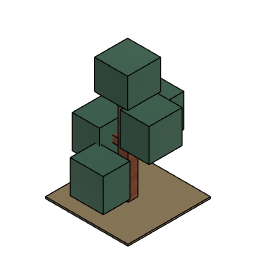
Tree v3 (Autodesk Fusion 360 design; units mm, degrees)
Autodesk Fusion 360 part; units mm, degrees
sketch "Skizze1" plane through (0, 0, 0) normal (0, 0, 1) x (1, 0, 0)
  line L0 (0, 0) -> (50, 0)
  line L1 (50, 0) -> (50, 50)
  line L2 (50, 50) -> (0, 50)
  line L3 (0, 50) -> (0, 0)
  line L4 (0, 25) -> (50, 25) construction
  line L5 (25, 50) -> (25, 0) construction
  constraint coincident L0.start L3.end
  constraint midpoint L3 L4.start
  constraint midpoint L1 L4.end
  constraint midpoint L2 L5.start
  constraint midpoint L0 L5.end
  constraint perpendicular L0 L5
extrude "Extrusion1" add sketch "Skizze1" against normal blind 1 makes body 1 in component "Ground"
ref_plane "Arbeitsebene1" through (25, 25, 0) normal (0, -1, 0) x (1, 0, 0)
ref_plane "Arbeitsebene2" through (25, 25, 0) normal (-1, 0, 0) x (0, -1, 0)
sketch "Skizze2" plane through (25, 25, 0) normal (0, -1, 0) x (1, 0, 0)
  line L0 (-25, 0) -> (25, 0)
  line L1 (0, 0) -> (0, 75) construction
  line L2 (-3, 0) -> (-3, 65)
  line L3 (-3, 65) -> (3, 65)
  line L4 (3, 65) -> (3, 0)
  line L5 (-3, 0) -> (3, 0)
  line L6 (-3, 29.6581) -> (-20.0867, 29.6581)
  line L7 (-20.0867, 29.6581) -> (-20.0867, 25.6581)
  line L8 (-20.0867, 25.6581) -> (-3, 25.6581)
  line L9 (-3, 25.6581) -> (-3, 29.6581)
  line L10 (3, 44.9151) -> (20.4397, 44.9151)
  line L11 (20.4397, 44.9151) -> (20.4397, 40.9151)
  line L12 (20.4397, 40.9151) -> (3, 40.9151)
  line L13 (3, 40.9151) -> (3, 44.9151)
  line L14 (-23.7757, 37.2774) -> (-7.2473, 37.2774)
  line L15 (-7.2473, 37.2774) -> (-7.2473, 17.2774)
  line L16 (-7.2473, 17.2774) -> (-23.7757, 17.2774)
  line L17 (-23.7757, 17.2774) -> (-23.7757, 37.2774)
  line L18 (5.3079, 53.1701) -> (22.7898, 53.1701)
  line L19 (22.7898, 53.1701) -> (22.7898, 33.1701)
  line L20 (22.7898, 33.1701) -> (5.3079, 33.1701)
  line L21 (5.3079, 33.1701) -> (5.3079, 53.1701)
  line L22 (-10.267, 73.036) -> (9.733, 73.036)
  line L23 (9.733, 73.036) -> (9.733, 55)
  line L24 (9.733, 55) -> (-10.267, 55)
  line L25 (-10.267, 55) -> (-10.267, 73.036)
  dimension "d21" = 6
  dimension "d25" = 3
  dimension "d26" = 4
  dimension "d27" = 4
  dimension "d36" = 20
  dimension "d37" = 20
  dimension "d38" = 20
  constraint coincident L1.start origin
  constraint perpendicular L0 L1
  constraint coincident L0 L2.start
  constraint perpendicular L0 L2
  constraint perpendicular L1 L3
  constraint coincident L0 L4.end
  constraint perpendicular L0 L4
  constraint horizontal L6
  constraint vertical L7
  constraint horizontal L8
  constraint vertical L9
  constraint coincident L2 L6.start
  constraint horizontal L10
  constraint vertical L11
  constraint horizontal L12
  constraint vertical L13
  constraint coincident L4 L10.start
  constraint horizontal L14
  constraint vertical L15
  constraint horizontal L16
  constraint vertical L17
  constraint horizontal L18
  constraint vertical L19
  constraint horizontal L20
  constraint vertical L21
  constraint horizontal L22
  constraint vertical L23
  constraint horizontal L24
  constraint vertical L25
  measures "d21" distance of L2.end L3.end
  measures "d25" distance of L1 L2
  measures "d26" distance of L6 L8
  measures "d27" distance of L10.end L11.end
  measures "d36" distance of L18.end L19.end
  measures "d37" distance of L14.start L16.end
  measures "d38" distance of L22.start L22.end
extrude "Extrusion1'" add sketch "Skizze2" along normal mid plane 6 separate body contours L0 L2 L4 L5 L9 L13 L24 | L2 L3 L4 L24 makes body 2 in component "Trunk"
sketch "Skizze3" plane through (25, 25, 0) normal (-1, 0, 0) x (0, 1, 0)
  line L0 (3, -65) -> (-3, -65)
  line L1 (-3, -65) -> (-3, 0)
  line L2 (-3, 0) -> (3, 0)
  line L3 (3, 0) -> (3, -65)
  line L4 (0, -44.9151) -> (0, -40.9151)
  line L5 (0, -29.6581) -> (0, -25.6581)
  line L6 (3, -40.2798) -> (19.6821, -40.2798)
  line L7 (19.6821, -40.2798) -> (19.6821, -36.2798)
  line L8 (19.6821, -36.2798) -> (3, -36.2798)
  line L9 (3, -36.2798) -> (3, -40.2798)
  line L10 (-3, -19.6193) -> (-20.4076, -19.6193)
  line L11 (-20.4076, -19.6193) -> (-20.4076, -15.6193)
  line L12 (-20.4076, -15.6193) -> (-3, -15.6193)
  line L13 (-3, -15.6193) -> (-3, -19.6193)
  line L14 (8.1625, -48.3226) -> (23.7982, -48.3226)
  line L15 (23.7982, -48.3226) -> (23.7982, -28.3226)
  line L16 (23.7982, -28.3226) -> (8.1625, -28.3226)
  line L17 (8.1625, -28.3226) -> (8.1625, -48.3226)
  line L18 (-25, -28.0196) -> (-8.8142, -28.0196)
  line L19 (-8.8142, -28.0196) -> (-8.8142, -8.0196)
  line L20 (-8.8142, -8.0196) -> (-25, -8.0196)
  line L21 (-25, -8.0196) -> (-25, -28.0196)
  line L22 (-20.4076, -17.6193) -> (-3, -17.6193) construction
  line L23 (3, -38.2798) -> (19.6821, -38.2798) construction
  dimension "d32" = 4
  dimension "d33" = 4
  dimension "d34" = 20
  dimension "d35" = 20
  constraint horizontal L6
  constraint vertical L7
  constraint horizontal L8
  constraint vertical L9
  constraint coincident L3 L6.start
  constraint horizontal L10
  constraint vertical L11
  constraint horizontal L12
  constraint vertical L13
  constraint coincident L1 L10.start
  constraint horizontal L14
  constraint vertical L15
  constraint horizontal L16
  constraint vertical L17
  constraint horizontal L18
  constraint vertical L19
  constraint horizontal L20
  constraint vertical L21
  constraint midpoint L11 L22.start
  constraint midpoint L13 L22.end
  constraint midpoint L9 L23.start
  constraint midpoint L7 L23.end
  measures "d32" distance of L10.end L11.end
  measures "d33" distance of L6.end L7.end
  measures "d34" distance of L18 L20
  measures "d35" distance of L14 L16
extrude "Extrusion1''" add sketch "Skizze3" along normal mid plane 4 separate body contours L3 L6 L8 L9 L17 | L1 L10 L12 L13 L19 | L6 L7 L8 L17 | L10 L11 L12 L19 makes body 3 at (24.3333, 10.395, 19.6193) makes body 4 at (23, 39.1214, 38.9465) in component "Branches Y"
extrude "Extrusion1'''" add sketch "Skizze2" along normal mid plane 4 separate body contours L2 L6 L8 L9 L15 | L4 L10 L12 L13 L21 | L6 L7 L8 L15 | L10 L11 L12 L21 makes body 5 at (10.6089, 24.3333, 25.6581) makes body 6 at (33.8132, 23, 42.2484) in component "Branches X"
extrude "Extrusion1''''" add sketch "Skizze2" along normal mid plane 20 separate body contours L6 L7 L8 L14 L15 L16 L17 | L6 L7 L8 L15 | L10 L11 L12 L21 | L10 L11 L12 L18 L19 L20 L21 | L2 L3 L4 L22 L23 L24 L25 | L2 L3 L4 L24 makes body 7 at (1.2243, 28.3333, 23.9441) makes body 8 at (30.3079, 28.3333, 39.8368) makes body 9 at (21.3997, 21.6667, 73.036) in component "Leaf X"
extrude "Extrusion1'''''" add sketch "Skizze3" along normal mid plane 20 separate body contours L6 L7 L8 L17 | L6 L7 L8 L14 L15 L16 L17 | L10 L11 L12 L18 L19 L20 L21 | L10 L11 L12 L19 makes body 10 at (28.3333, 16.1858, 21.3529) makes body 11 at (21.6667, 33.1625, 41.656) in component "Leaf Y"
component "Ground" placed x (1, 0, 0) y (0, 1, 0) z (0, 0, 1) at (0, 0, 0)
component "Trunk" placed x (1, 0, 0) y (0, 1, 0) z (0, 0, 1) at (0, 0, 0)
component "Branches Y" placed x (1, 0, 0) y (0, 1, 0) z (0, 0, 1) at (0, 0, 0)
component "Branches X" placed x (1, 0, 0) y (0, 1, 0) z (0, 0, 1) at (0, 0, 0)
component "Leaf X" placed x (1, 0, 0) y (0, 1, 0) z (0, 0, 1) at (0, 0, 0)
component "Leaf Y" placed x (1, 0, 0) y (0, 1, 0) z (0, 0, 1) at (0, 0, 0)
equation "d21 = d_trunk"
equation "d_trunk = 6 mm" comment "Diameter Treetrunk"
equation "d_branch = 4 mm" comment "Diameter tree branch"
equation "d_leaf = 20 mm" comment "diameter leafball"
equation "d25 = d21 / 2"
equation "d26 = d_branch"
equation "d27 = d_branch"
equation "d30 = d_trunk / 2"
equation "d32 = d_branch"
equation "d33 = d_branch"
equation "d34 = d_leaf"
equation "d35 = d_leaf"
equation "d36 = d_leaf"
equation "d37 = d_leaf"
equation "d38 = d_leaf"
equation "d39 = d_branch / 2"
equation "d41 = d_branch / 2"
equation "d43 = d_leaf / 2"
equation "d45 = d_leaf / 2"
